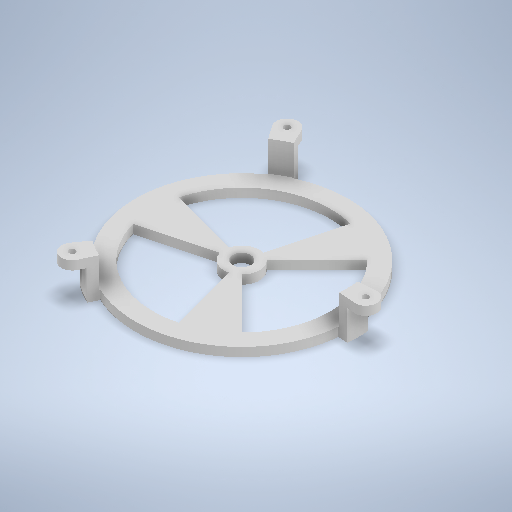
# Autodesk Inventor part: MechSwitch_DielecTop
Saved by Autodesk Inventor 2025.1 (Build 291241000, 241)
## iProperties
Created: 2026-02-23
Part Number: MechSwitch_DielecTop
Material: Generic
Document SubType Name: Modeling
Designer: ryand
Density: 1 g/cm^3
Appearance: Default
Author: ryand
Autodesk Inventor part; units mm, degrees
ref_plane "YZ Plane" through (0, 0, 0) normal (1, 0, 0) x (0, 1, 0)
ref_plane "XZ Plane" through (0, 0, 0) normal (0, 1, 0) x (-1, 0, 0)
ref_plane "XY Plane" through (0, 0, 0) normal (0, 0, 1) x (1, 0, 0)
sketch "Sketch1" plane through (0, 0, 0) normal (0, 1, 0) x (-1, 0, 0)
  line L0 (0, 0) -> (48.2963, -12.941)
  line L1 (0, 0) -> (50, 0) construction
  line L2 (0, 0) -> (48.2963, 12.941)
  line L3 (0, 0) -> (50, 0) construction
  arc A0 (48.2963, -12.941) -> (48.2963, 12.941) centre (0, 0) ccw
  arc A1 (-12.941, 48.2963) -> (-35.3553, 35.3553) centre (0, 0) ccw
  line L4 (0, 0) -> (-12.941, 48.2963)
  line L5 (0, 0) -> (-35.3553, 35.3553)
  arc A2 (-35.3553, -35.3553) -> (-12.941, -48.2963) centre (0, 0) ccw
  line L6 (0, 0) -> (-35.3553, -35.3553)
  line L7 (0, 0) -> (-12.941, -48.2963)
  circle A3 centre (0, 0) radius 5
  circle A4 centre (0, 0) radius 10
  line L8 (0, 0) -> (34.7014, -49.5587)
  line L9 (0, 0) -> (60.5, 0) construction
  line L10 (0, 0) -> (25.5684, -54.8316)
  line L11 (0, 0) -> (60.5, 0) construction
  line L12 (25.5684, -54.8316) -> (27.6815, -59.3632)
  line L13 (34.7014, -49.5587) -> (37.5693, -53.6545)
  arc A5 (27.6815, -59.3632) -> (37.5693, -53.6545) centre (0, 0) ccw
  circle A6 centre (0, 0) radius 50
  circle A7 centre (0, 0) radius 60
  line L14 (0, 0) -> (25.5684, 54.8316)
  line L15 (25.5684, 54.8316) -> (27.6815, 59.3632)
  arc A8 (37.5693, 53.6545) -> (27.6815, 59.3632) centre (0, 0) ccw
  line L16 (0, 0) -> (34.7014, 49.5587)
  line L17 (34.7014, 49.5587) -> (37.5693, 53.6545)
  line L18 (0, 0) -> (-60.2698, -5.2729)
  line L19 (-60.2698, -5.2729) -> (-65.2508, -5.7087)
  arc A9 (-65.2508, 5.7087) -> (-65.2508, -5.7087) centre (0, 0) ccw
  line L20 (0, 0) -> (-60.2698, 5.2729)
  line L21 (-60.2698, 5.2729) -> (-65.2508, 5.7087)
  point P0 (9.6593, -2.5882)
  point P1 (9.6593, 2.5882)
  point P2 (-2.5882, 9.6593)
  point P3 (-7.0711, 7.0711)
  point P4 (-7.0711, -7.0711)
  point P5 (-2.5882, -9.6593)
  point P6 (4.2262, -9.0631)
  point P7 (5.7358, -8.1915)
  point P8 (-35.3553, -35.3553)
  point P9 (-35.3553, 35.3553)
  point P10 (-12.941, 48.2963)
  point P11 (-12.941, -48.2963)
  point P12 (25.3571, -54.3785)
  point P13 (34.4146, -49.1491)
  point P14 (34.4146, 49.1491)
  point P15 (25.3571, 54.3785)
  point P16 (-59.7717, 5.2293)
  point P17 (-59.7717, -5.2293)
  dimension "d0" = 50
  dimension "d1" = 15
  dimension "d2" = 50
  dimension "d3" = 15
  dimension "d4" = 50
  dimension "d7" = 360
  dimension "d9" = 10
  dimension "d10" = 20
  dimension "d11" = 60.5
  dimension "d12" = 55
  dimension "d13" = 60.5
  dimension "d14" = 65
  dimension "d16" = 5
  dimension "d17" = 5
  dimension "d18" = 65.5
  dimension "d25" = 100
  dimension "d26" = 120
  dimension "d29" = 360
  constraints: 44 end point, 12 point on circle, 10 centre point, 6 coincident, 4 equal length, 4 horizontal, 54 other
  measures "d0" distance of L0.start L0.end
  measures "d1" angle of L0 L1
  measures "d2" distance of L0.start L2.end
  measures "d3" angle of L3 L2
  measures "d4" radius of A0
  measures "d9" diameter of A3
  measures "d10" diameter of A4
  measures "d11" distance of L8.start L8.end
  measures "d12" angle of L8 L9
  measures "d13" distance of L8.start L10.end
  measures "d14" angle of L10 L11
  measures "d16" distance of L10.end L12.end
  measures "d17" distance of L8.end L13.end
  measures "d18" radius of A5
  measures "d25" diameter of A6
  measures "d26" diameter of A7
extrude "Extrusion2" add sketch "Sketch1" along normal blind 5 contours A3 L2 A4 L0 | L0 A4 L8 A3 | A3 L16 A4 L2 | A3 L5 A4 L4 | L4 A4 L14 A3 | A3 L20 A4 L5 | A3 L7 A4 L6 | L6 A4 L18 A3 | A3 L10 A4 L7 | L8 A4 L10 A3 | L14 A4 L16 A3 | L18 A4 L20 A3 | A4 L2 A0 L0 | A4 L5 A1 L4 | A4 L7 A2 L6 | A0 A6 L16 A7 L8 | A1 A6 L20 A7 L14 | A2 A6 L10 A7 L18 | L8 A7 L10 A6 | L14 A7 L16 A6 | L18 A7 L20 A6 | L8 L13 A5 L12 L10 A7 | L14 L15 A8 L17 L16 A7 | L18 L19 A9 L21 L20 A7
sketch "Sketch3" plane through (0, 5, 0) normal (0, 1, 0) x (1, 0, 0)
  circle A0 centre (0, 0) radius 5 projected
  arc A1 (65.2508, -5.7087) -> (65.2508, 5.7087) centre (0, 0) ccw projected
  arc A2 (65.2508, -5.7087) -> (65.2508, 5.7087) centre (0, 0) ccw
  line L0 (65.2508, 5.7087) -> (60.2698, 5.2729)
  line L1 (65.2508, 5.7087) -> (59.7717, 5.2293) projected
  line L2 (65.2508, -5.7087) -> (60.2698, -5.2729)
  line L3 (59.7717, -5.2293) -> (65.2508, -5.7087) projected
  arc A3 (60.2698, -5.2729) -> (60.2698, 5.2729) centre (0, 0) ccw
  arc A4 (-27.6815, 59.3632) -> (-37.5693, 53.6545) centre (0, 0) ccw
  line L4 (-37.5693, 53.6545) -> (-34.7014, 49.5587)
  arc A5 (-25.5684, 54.8316) -> (-34.7014, 49.5587) centre (0, 0) ccw
  line L5 (-27.6815, 59.3632) -> (-25.5684, 54.8316)
  arc A6 (-37.5693, -53.6545) -> (-27.6815, -59.3632) centre (0, 0) ccw
  line L6 (-27.6815, -59.3632) -> (-25.5684, -54.8316)
  arc A7 (-34.7014, -49.5587) -> (-25.5684, -54.8316) centre (0, 0) ccw
  line L7 (-37.5693, -53.6545) -> (-34.7014, -49.5587)
  dimension "d40" = 5
  dimension "d41" = 5
  dimension "d42" = 60.5
  dimension "d45" = 360
  constraints: 12 end point, 12 point on circle, 6 centre point, 2 point on line, 1 coincident, 31 other
  measures "d40" distance of L0.start L0.end
  measures "d41" distance of L2.start L2.end
  measures "d42" radius of A3
extrude "Extrusion3" add sketch "Sketch3" along normal blind 17 contours L2 A3 L0 A1 | L5 A5 L4 A4 | L7 A7 L6 A6
sketch "Sketch4" plane through (0, 22, 0) normal (0, 1, 0) x (1, 0, 0)
  arc A0 (-27.6815, 59.3632) -> (-37.5693, 53.6545) centre (0, 0) ccw projected
  arc A1 (-27.6815, 59.3632) -> (-37.5693, 53.6545) centre (0, 0) ccw
  line L0 (-27.6815, 59.3632) -> (-29.5833, 63.4415)
  line L1 (-27.6815, 59.3632) -> (-23.1815, 59.3632) construction
  line L2 (-37.5693, 53.6545) -> (-40.1504, 57.3406)
  line L3 (-37.5693, 53.6545) -> (-33.0693, 53.6545) construction
  circle A2 centre (-35, 60.6218) radius 1.75
  arc A3 (-29.5833, 63.4415) -> (-40.1504, 57.3406) centre (-35, 60.6218) ccw
  arc A4 (-40.1504, -57.3406) -> (-29.5833, -63.4415) centre (-35, -60.6218) ccw
  circle A5 centre (-35, -60.6218) radius 1.75
  line L4 (-37.5693, -53.6545) -> (-40.1504, -57.3406)
  line L5 (-27.6815, -59.3632) -> (-29.5833, -63.4415)
  arc A6 (-37.5693, -53.6545) -> (-27.6815, -59.3632) centre (0, 0) ccw
  arc A7 (69.7336, -6.1009) -> (69.7336, 6.1009) centre (70, 0) ccw
  circle A8 centre (70, 0) radius 1.75
  line L6 (65.2508, -5.7087) -> (69.7336, -6.1009)
  line L7 (65.2508, 5.7087) -> (69.7336, 6.1009)
  arc A9 (65.2508, -5.7087) -> (65.2508, 5.7087) centre (0, 0) ccw
  point P0 (0, 0)
  dimension "d50" = 4.5
  dimension "d51" = 115
  dimension "d52" = 4.5
  dimension "d53" = 125
  dimension "d63" = 3.5
  dimension "d66" = 360
  dimension "d70" = 70
  constraints: 16 end point, 12 point on circle, 9 centre point, 5 coincident, 2 equal length, 2 horizontal, 35 other
  measures "d50" distance of L0.start L0.end
  measures "d51" angle of L1 L0
  measures "d52" distance of L2.start L2.end
  measures "d53" angle of L3 L2
  measures "d63" diameter of A2
  measures "d70" distance of A7.centre A0.centre
extrude "Extrusion5" add sketch "Sketch4" against normal blind 5
body "Solid2"
